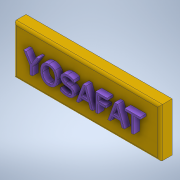
# Autodesk Inventor part: Repujado 1
Saved by Autodesk Inventor 2021 (Build 250183000, 183)
## iProperties
Created: 2021-01-13
Part Number: Repujado 1
Material: Genérico
Document SubType Name: Modeling
Designer: yosaf
Density: 1 g/cm^3
Appearance: Valor por defecto
Author: yosaf
Autodesk Inventor part; units mm, degrees
ref_plane "YZ Plane" through (0, 0, 0) normal (1, 0, 0) x (0, 1, 0)
ref_plane "XZ Plane" through (0, 0, 0) normal (0, 1, 0) x (-1, 0, 0)
sketch "Boceto1" plane through (0, 0, 0) normal (0, 0, 1) x (1, 0, 0)
  line L0 (0, 0) -> (-60, 0) construction
  line L1 (-60, 0) -> (-60, 20) construction
  line L2 (-60, 20) -> (60, 20)
  line L3 (60, 20) -> (60, -20)
  line L4 (60, -20) -> (-60, -20)
  line L5 (-60, -20) -> (-60, 20)
  dimension "d0" = 60
  dimension "d1" = 20
  dimension "d2" = 120
  dimension "d3" = 40
  constraints: 12 end point, 2 horizontal, 2 parallel, 2 perpendicular
  measures "d0" distance of L0.start L0.end
  measures "d1" distance of L0.end L1.end
  measures "d2" distance of L3.end L4.end
  measures "d3" distance of L2.end L3.end
extrude "Extrusión1" add sketch "Boceto1" along normal blind 10
fillet "Empalme1" radius 2 4 edges at (0, 20, 10) (60, 0, 10) (0, -20, 10) (-60, 0, 10)
ref_plane "Plano de trabajo1" through (0, 0, 10) normal (0, 0, 1) x (1, 0, 0)
sketch "Boceto2" plane through (0, 0, 10) normal (0, 0, 1) x (1, 0, 0)
  line L0 (-47.1397, 9.0462) -> (47.4717, 9.0462) construction
  line L1 (47.4717, 9.0462) -> (47.4717, -9.0462) construction
  line L2 (47.4717, -9.0462) -> (-47.1397, -9.0462) construction
  line L3 (-47.1397, -9.0462) -> (-47.1397, 9.0462) construction
  line L4 (-60, 20) -> (-60, -20) construction
  line L5 (-60, 0) -> (-47.3055, 0) construction
  line L6 (60, -20) -> (60, 20) construction
  line L7 (-34.503, 8.7278) -> (-39.7806, 0.3033)
  line L8 (-39.7806, 0.3033) -> (-39.7806, -6.2722)
  line L9 (-39.7806, -6.2722) -> (-41.7765, -6.2722)
  line L10 (-41.7765, -6.2722) -> (-41.7765, 0.0952)
  line L11 (-41.7765, 0.0952) -> (-47.0785, 8.7278)
  line L12 (-47.0785, 8.7278) -> (-44.8622, 8.7278)
  line L13 (-44.8622, 8.7278) -> (-40.7724, 2.0176)
  line L14 (-40.7724, 2.0176) -> (-36.6214, 8.7278)
  line L15 (-36.6214, 8.7278) -> (-34.503, 8.7278)
  spline S0 degree 2 poles (-21.254, 7.0135) (-20.3357, 5.9972) (-19.3561, 3.0829) (-19.3561, 1.2217) knots 0 0 0 1 2 2 2
  spline S1 degree 2 poles (-19.3561, 1.2217) (-19.3561, -0.6273) (-20.3479, -3.5661) (-21.254, -4.5457) knots 0 0 0 1 2 2 2
  spline S2 degree 2 poles (-21.254, -4.5457) (-22.1724, -5.562) (-24.7071, -6.5906) (-26.3234, -6.5906) knots 0 0 0 1 2 2 2
  spline S3 degree 2 poles (-26.3234, -6.5906) (-27.903, -6.5906) (-30.4867, -5.5375) (-31.3928, -4.5457) knots 0 0 0 1 2 2 2
  spline S4 degree 2 poles (-31.3928, -4.5457) (-32.2989, -3.5416) (-33.2785, -0.6395) (-33.2785, 1.2217) knots 0 0 0 1 2 2 2
  spline S5 degree 2 poles (-33.2785, 1.2217) (-33.2785, 3.0584) (-32.3112, 5.9727) (-31.3806, 7.0135) knots 0 0 0 1 2 2 2
  spline S6 degree 2 poles (-31.3806, 7.0135) (-30.4989, 7.9931) (-27.8785, 9.0462) (-26.3234, 9.0462) knots 0 0 0 1 2 2 2
  spline S7 degree 2 poles (-26.3234, 9.0462) (-24.7071, 9.0462) (-22.1479, 7.9931) (-21.254, 7.0135) knots 0 0 0 1 2 2 2
  spline S8 degree 2 poles (-21.4254, 1.2217) (-21.4254, 4.1482) (-24.0459, 7.3197) (-26.3112, 7.3197) knots 0 0 0 1 2 2 2
  spline S9 degree 2 poles (-26.3112, 7.3197) (-28.601, 7.3197) (-31.2091, 4.1482) (-31.2091, 1.2217) knots 0 0 0 1 2 2 2
  spline S10 degree 2 poles (-31.2091, 1.2217) (-31.2091, -1.7293) (-28.552, -4.864) (-26.3112, -4.864) knots 0 0 0 1 2 2 2
  spline S11 degree 2 poles (-26.3112, -4.864) (-24.0703, -4.864) (-21.4254, -1.7293) (-21.4254, 1.2217) knots 0 0 0 1 2 2 2
  spline S12 degree 2 poles (-5.2867, -1.9865) (-5.2867, -2.8681) (-6.1071, -4.5824) (-6.8418, -5.1701) knots 0 0 0 1 2 2 2
  spline S13 degree 2 poles (-6.8418, -5.1701) (-7.6499, -5.8191) (-9.7928, -6.5416) (-11.2989, -6.5416) knots 0 0 0 1 2 2 2
  spline S14 degree 2 poles (-11.2989, -6.5416) (-12.9275, -6.5416) (-15.5234, -5.9416) (-16.8581, -5.3416) knots 0 0 0 1 2 2 2
  line L16 (-16.8581, -5.3416) -> (-16.8581, -2.8436)
  line L17 (-16.8581, -2.8436) -> (-16.7112, -2.8436)
  spline S15 degree 2 poles (-16.7112, -2.8436) (-15.5724, -3.7865) (-12.5969, -4.815) (-11.2744, -4.815) knots 0 0 0 1 2 2 2
  spline S16 degree 2 poles (-11.2744, -4.815) (-9.4254, -4.815) (-7.3561, -3.4314) (-7.3561, -2.2681) knots 0 0 0 1 2 2 2
  spline S17 degree 2 poles (-7.3561, -2.2681) (-7.3561, -1.2763) (-8.3357, -0.3334) (-9.3397, -0.064) knots 0 0 0 1 2 2 2
  spline S18 degree 2 poles (-9.3397, -0.064) (-10.0867, 0.1319) (-11.8622, 0.4013) (-12.8418, 0.5972) knots 0 0 0 1 2 2 2
  spline S19 degree 2 poles (-12.8418, 0.5972) (-14.8499, 1.0258) (-16.7724, 3.0707) (-16.7724, 4.7115) knots 0 0 0 1 2 2 2
  spline S20 degree 2 poles (-16.7724, 4.7115) (-16.7724, 6.585) (-13.5887, 8.9972) (-11.1275, 8.9972) knots 0 0 0 1 2 2 2
  spline S21 degree 2 poles (-11.1275, 8.9972) (-9.5479, 8.9972) (-6.903, 8.3972) (-5.8867, 7.9441) knots 0 0 0 1 2 2 2
  line L18 (-5.8867, 7.9441) -> (-5.8867, 5.5931)
  line L19 (-5.8867, 5.5931) -> (-6.0336, 5.5931)
  spline S22 degree 2 poles (-6.0336, 5.5931) (-6.8908, 6.3156) (-9.6826, 7.2707) (-11.152, 7.2707) knots 0 0 0 1 2 2 2
  spline S23 degree 2 poles (-11.152, 7.2707) (-12.7561, 7.2707) (-14.703, 5.9482) (-14.703, 4.8952) knots 0 0 0 1 2 2 2
  spline S24 degree 2 poles (-14.703, 4.8952) (-14.703, 3.9645) (-13.7357, 2.8992) (-12.5112, 2.6176) knots 0 0 0 1 2 2 2
  spline S25 degree 2 poles (-12.5112, 2.6176) (-11.8622, 2.4707) (-9.4867, 2.0666) (-8.654, 1.8584) knots 0 0 0 1 2 2 2
  spline S26 degree 2 poles (-8.654, 1.8584) (-6.9765, 1.4176) (-5.2867, -0.3824) (-5.2867, -1.9865) knots 0 0 0 1 2 2 2
  line L20 (9.7501, -6.2722) -> (7.6317, -6.2722)
  line L21 (7.6317, -6.2722) -> (6.1623, -2.1089)
  line L22 (6.1623, -2.1089) -> (-0.3642, -2.1089)
  line L23 (-0.3642, -2.1089) -> (-1.8214, -6.2722)
  line L24 (-1.8214, -6.2722) -> (-3.8418, -6.2722)
  line L25 (-3.8418, -6.2722) -> (1.6194, 8.7278)
  line L26 (1.6194, 8.7278) -> (4.2888, 8.7278)
  line L27 (4.2888, 8.7278) -> (9.7501, -6.2722)
  line L28 (5.5378, -0.3824) -> (2.9052, 6.989)
  line L29 (2.9052, 6.989) -> (0.2603, -0.3824)
  line L30 (0.2603, -0.3824) -> (5.5378, -0.3824)
  line L31 (21.6031, 6.9523) -> (14.0235, 6.9523)
  line L32 (14.0235, 6.9523) -> (14.0235, 2.7278)
  line L33 (14.0235, 2.7278) -> (20.5378, 2.7278)
  line L34 (20.5378, 2.7278) -> (20.5378, 0.9523)
  line L35 (20.5378, 0.9523) -> (14.0235, 0.9523)
  line L36 (14.0235, 0.9523) -> (14.0235, -6.2722)
  line L37 (14.0235, -6.2722) -> (12.0276, -6.2722)
  line L38 (12.0276, -6.2722) -> (12.0276, 8.7278)
  line L39 (12.0276, 8.7278) -> (21.6031, 8.7278)
  line L40 (21.6031, 8.7278) -> (21.6031, 6.9523)
  line L41 (35.7092, -6.2722) -> (33.5909, -6.2722)
  line L42 (33.5909, -6.2722) -> (32.1215, -2.1089)
  line L43 (32.1215, -2.1089) -> (25.595, -2.1089)
  line L44 (25.595, -2.1089) -> (24.1378, -6.2722)
  line L45 (24.1378, -6.2722) -> (22.1174, -6.2722)
  line L46 (22.1174, -6.2722) -> (27.5786, 8.7278)
  line L47 (27.5786, 8.7278) -> (30.248, 8.7278)
  line L48 (30.248, 8.7278) -> (35.7092, -6.2722)
  line L49 (31.497, -0.3824) -> (28.8643, 6.989)
  line L50 (28.8643, 6.989) -> (26.2194, -0.3824)
  line L51 (26.2194, -0.3824) -> (31.497, -0.3824)
  line L52 (48.6888, 6.9523) -> (43.3256, 6.9523)
  line L53 (43.3256, 6.9523) -> (43.3256, -6.2722)
  line L54 (43.3256, -6.2722) -> (41.3297, -6.2722)
  line L55 (41.3297, -6.2722) -> (41.3297, 6.9523)
  line L56 (41.3297, 6.9523) -> (35.9664, 6.9523)
  line L57 (35.9664, 6.9523) -> (35.9664, 8.7278)
  line L58 (35.9664, 8.7278) -> (48.6888, 8.7278)
  line L59 (48.6888, 8.7278) -> (48.6888, 6.9523)
  point P0 (0, 0)
  dimension "d8" = 94.6114
  dimension "d9" = 12.6945
  dimension "d10" = 12.5283
  constraints: 2 end point, 1 horizontal, 1 midpoint, 2 other
  measures "d8" distance of L0.end L0.start
  measures "d9" distance of L5.start L5.end
  measures "d10" distance between parallel lines of L6 L1
extrude "Extrusión2" add sketch "Boceto2" along normal blind 5
